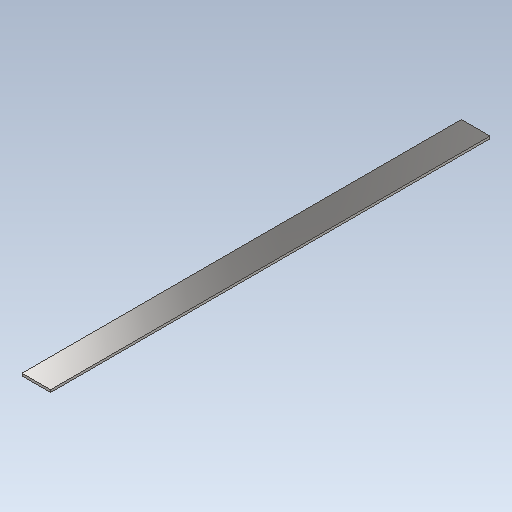
# Autodesk Inventor part: Lift.03.01.00.03
Saved by Autodesk Inventor 2021 (Build 250183000, 183)
## iProperties
Created: 2020-09-20
Part Number: Lift.03.01.00.03
Material: Сталь нержавеющая, 440C
Document SubType Name: ЛистМат
Designer: Kostya
Density: 7.75 g/cm^3
Sheet Metal Rule: По умолчанию_мм
Appearance: С умеренной полировкой
Author: Kostya
Autodesk Inventor part; units mm, degrees
ref_plane "YZ Plane" through (0, 0, 0) normal (1, 0, 0) x (0, 1, 0)
ref_plane "XZ Plane" through (0, 0, 0) normal (0, 1, 0) x (-1, 0, 0)
ref_plane "XY Plane" through (0, 0, 0) normal (0, 0, 1) x (1, 0, 0)
sketch "Эскиз1" plane through (0, 0, 0) normal (0, 1, 0) x (-1, 0, 0)
  line L0 (-60, -922.5) -> (60, -922.5)
  line L1 (60, -922.5) -> (60, 922.5)
  line L2 (60, 922.5) -> (-60, 922.5)
  line L3 (-60, 922.5) -> (-60, -922.5)
  line L4 (-60, -922.5) -> (60, 922.5) construction
  line L5 (60, -922.5) -> (-60, 922.5) construction
  point P0 (0, 0)
  dimension "d0" = 120
  dimension "d1" = 1845
  measures "d0" distance of L2.end L1.end
  measures "d1" distance of L1.end L0.end
extrude "Пластина1" add sketch "Эскиз1" along normal blind 10
equation "\"d2\" = Толщина"
equation "\"Глубина_просечки\" = 0.5 * Толщина"
equation "\"Толщина\" = 10"
